Autodesk Fusion 360 part; units mm, degrees
note: some values were not read from the file. Chosen so that the rebuilt part matches the saved one: that a step has no effect.
(part 7 of 7)
  spline S315 degree 3 poles (62.2159, 94.3594) (61.6701, 95.351) (61.6701, 95.351) (61.5911, 95.6457) knots 0 0 0 0 1 1 1 1
  spline S316 degree 3 poles (61.5911, 95.6457) (61.8402, 95.8709) (62.0898, 96.0953) (62.3397, 96.3195) knots 0 0 0 0 1 1 1 1
  spline S317 degree 3 poles (62.3397, 96.3195) (62.4451, 96.4149) (62.4451, 96.4149) (62.5526, 96.5123) knots 0 0 0 0 1 1 1 1
  spline S318 degree 3 poles (62.5526, 96.5123) (63.3308, 97.2082) (64.2415, 97.7243) (65.322, 97.5831) knots 0 0 0 0 1 1 1 1
  spline S319 degree 3 poles (-22.0549, 83.1437) (-21.9278, 83.1778) (-21.8007, 83.2119) (-21.6697, 83.247) knots 0 0 0 0 1 1 1 1
  spline S320 degree 3 poles (-21.6697, 83.247) (-21.2763, 82.8034) (-21.2052, 82.1251) (-21.0547, 81.5621) knots 0 0 0 0 1 1 1 1
  spline S321 degree 3 poles (-21.0547, 81.5621) (-21.0162, 81.4183) (-20.9777, 81.2746) (-20.938, 81.1265) knots 0 0 0 0 1 1 1 1
  spline S322 degree 3 poles (-20.938, 81.1265) (-20.5691, 79.7113) (-20.212, 78.2272) (-20.2059, 76.7566) knots 0 0 0 0 1 1 1 1
  spline S323 degree 3 poles (-20.2059, 76.7566) (-21.5811, 76.4463) (-22.956, 76.389) (-24.3593, 76.332) knots 0 0 0 0 1 1 1 1
  spline S324 degree 3 poles (-24.3593, 76.332) (-24.1584, 77.2005) (-23.9104, 78.0286) (-23.5915, 78.8606) knots 0 0 0 0 1 1 1 1
  spline S325 degree 3 poles (-23.5915, 78.8606) (-23.3151, 79.5912) (-23.0456, 80.3225) (-22.7959, 81.0627) knots 0 0 0 0 1 1 1 1
  spline S326 degree 3 poles (-22.7959, 81.0627) (-22.7509, 81.195) (-22.706, 81.3273) (-22.6597, 81.4636) knots 0 0 0 0 1 1 1 1
  spline S327 degree 3 poles (-22.6597, 81.4636) (-22.5724, 81.7219) (-22.4863, 81.9806) (-22.4015, 82.2397) knots 0 0 0 0 1 1 1 1
  spline S328 degree 3 poles (-22.4015, 82.2397) (-22.3618, 82.3564) (-22.3221, 82.4731) (-22.2812, 82.5933) knots 0 0 0 0 1 1 1 1
  spline S329 degree 3 poles (-22.2812, 82.5933) (-22.2295, 82.7492) (-22.2295, 82.7492) (-22.1768, 82.9082) knots 0 0 0 0 1 1 1 1
  spline S330 degree 3 poles (-22.1768, 82.9082) (-22.1366, 82.9859) (-22.0964, 83.0636) (-22.0549, 83.1437) knots 0 0 0 0 1 1 1 1
  spline S331 degree 3 poles (61.5057, 102.6431) (61.936, 102.5114) (62.1851, 102.4146) (62.4827, 102.0789) knots 0 0 0 0 1 1 1 1
  spline S332 degree 3 poles (62.4827, 102.0789) (62.7043, 101.4281) (62.7203, 100.8901) (62.4367, 100.2599) knots 0 0 0 0 1 1 1 1
  spline S333 degree 3 poles (62.4367, 100.2599) (61.9549, 99.393) (61.2756, 98.5426) (60.3891, 98.0767) knots 0 0 0 0 1 1 1 1
  spline S334 degree 3 poles (60.3891, 98.0767) (60.05, 98.4814) (59.7123, 98.8872) (59.3749, 99.2933) knots 0 0 0 0 1 1 1 1
  spline S335 degree 3 poles (59.3749, 99.2933) (59.2784, 99.4084) (59.1819, 99.5235) (59.0825, 99.6421) knots 0 0 0 0 1 1 1 1
  spline S336 degree 3 poles (59.0825, 99.6421) (58.9907, 99.7528) (58.8989, 99.8635) (58.8044, 99.9776) knots 0 0 0 0 1 1 1 1
  spline S337 degree 3 poles (58.8044, 99.9776) (58.7194, 100.0795) (58.6344, 100.1815) (58.5468, 100.2865) knots 0 0 0 0 1 1 1 1
  spline S338 degree 3 poles (58.5468, 100.2865) (58.3477, 100.558) (58.3477, 100.558) (58.2445, 100.9433) knots 0 0 0 0 1 1 1 1
  spline S339 degree 3 poles (58.2445, 100.9433) (58.57, 101.1706) (58.8969, 101.3953) (59.2249, 101.619) knots 0 0 0 0 1 1 1 1
  spline S340 degree 3 poles (59.2249, 101.619) (59.361, 101.7145) (59.361, 101.7145) (59.4998, 101.812) knots 0 0 0 0 1 1 1 1
  spline S341 degree 3 poles (59.4998, 101.812) (60.1264, 102.2358) (60.7438, 102.5566) (61.5057, 102.6431) knots 0 0 0 0 1 1 1 1
extrude "Extrude6" cut sketch "Sketch107" against normal blind 0.4 contours S0 S1 S2 S3 S4 S5 S6 S7 S8 S9 S10 S11 S12 S13 S14 S15 S16 S17 S18 S19 S20 S21 S22 S23 S24 S25 S26 S27 S28 S29 S30 S31 S32 S33 S34 S35 S36 S37 S38 S39 S40 S41 S42 S43 S44 S45 S46 S47 S48 S49 S50 S51 S52 S53 S54 S65 S66 S67 S114 S115 S116 S117 S118 S119 S120 | S54 S55 S56 S57 S58 S59 S60 S61 S62 S63 S64 S65 S114 S115 S116 S117 S118 S119 S120 S121 S122 S123 S124 S125 S126 S127 S128 S129 S130 | S308 S309 S310 S311 S312 S313 S314 S315 S316 S317 S318 | S319 S320 S321 S322 S323 S324 S325 S326 S327 S328 S329 S330 | S331 S332 S333 S334 S335 S336 S337 S338 S339 S340 S341 bodies 2 in component "Component"
sketch "Sketch108" plane through (0, -33.2802, 118.858) normal (0, -0.26963, 0.962964) x (1, 0, 0)
  line L0 (-103.3594, -20.3608) -> (76.6406, -20.3608)
  line L1 (76.6406, -20.3608) -> (76.6406, 97.166)
  line L2 (76.6406, 97.166) -> (71.6406, 97.166)
  line L3 (71.6406, 97.166) -> (71.6406, 62.066)
  line L4 (71.6406, 62.066) -> (-98.3594, 62.066)
  line L5 (-98.3594, 62.066) -> (-98.3594, 97.166)
  line L6 (-98.3594, 97.166) -> (-103.3594, 97.166)
  line L7 (-103.3594, 97.166) -> (-103.3594, -20.3608)
  spline S0 degree 3 poles (-85.2606, 64.3178) (-39.3625, 64.3178) (6.5356, 64.3178) (53.8246, 64.3178) knots 0 0 0 0 1 1 1 1
  spline S1 degree 3 poles (53.8246, 64.3178) (53.8246, 35.1839) (53.8246, 6.05) (53.8246, -23.9668) knots 0 0 0 0 1 1 1 1
  spline S2 degree 3 poles (53.8246, -23.9668) (7.9265, -23.9668) (-37.9717, -23.9668) (-85.2606, -23.9668) knots 0 0 0 0 1 1 1 1
  spline S3 degree 3 poles (-85.2606, -23.9668) (-85.2606, 5.1671) (-85.2606, 34.3011) (-85.2606, 64.3178) knots 0 0 0 0 1 1 1 1
  spline S4 degree 3 poles (-40.7041, 45.5277) (-42.4517, 43.0465) (-42.7552, 40.6645) (-42.3514, 37.6845) knots 0 0 0 0 1 1 1 1
  spline S5 degree 3 poles (-42.3514, 37.6845) (-41.6687, 35.5957) (-40.6171, 34.2385) (-38.7448, 33.0915) knots 0 0 0 0 1 1 1 1
  spline S6 degree 3 poles (-38.7448, 33.0915) (-35.2679, 31.3825) (-32.3234, 31.0033) (-28.5415, 31.766) knots 0 0 0 0 1 1 1 1
  spline S7 degree 3 poles (-28.5415, 31.766) (-26.5081, 32.5567) (-24.9395, 33.4626) (-23.6094, 35.2184) knots 0 0 0 0 1 1 1 1
  spline S8 degree 3 poles (-23.6094, 35.2184) (-23.6767, 36.3127) (-23.6767, 36.3127) (-24.1026, 37.1913) knots 0 0 0 0 1 1 1 1
  spline S9 degree 3 poles (-24.1026, 37.1913) (-25.7404, 37.0008) (-26.8845, 36.8089) (-28.2949, 35.9274) knots 0 0 0 0 1 1 1 1
  spline S10 degree 3 poles (-28.2949, 35.9274) (-29.8328, 35.0431) (-30.7377, 34.9951) (-32.4872, 35.2184) knots 0 0 0 0 1 1 1 1
  spline S11 degree 3 poles (-32.4872, 35.2184) (-34.0338, 36.0963) (-34.3816, 36.4628) (-34.9532, 38.1777) knots 0 0 0 0 1 1 1 1
  spline S12 degree 3 poles (-34.9532, 38.1777) (-35.2257, 40.9021) (-34.6294, 42.6777) (-33.4601, 45.0749) knots 0 0 0 0 1 1 1 1
  spline S13 degree 3 poles (-33.4601, 45.0749) (-32.9256, 46.1286) (-32.9256, 46.1286) (-32.4872, 47.5487) knots 0 0 0 0 1 1 1 1
  spline S14 degree 3 poles (-32.4872, 47.5487) (-31.7786, 47.5888) (-31.0695, 47.6174) (-30.3602, 47.6412) knots 0 0 0 0 1 1 1 1
  spline S15 degree 3 poles (-30.3602, 47.6412) (-29.768, 47.6669) (-29.768, 47.6669) (-29.1638, 47.6932) knots 0 0 0 0 1 1 1 1
  spline S16 degree 3 poles (-29.1638, 47.6932) (-27.7795, 47.5139) (-27.4143, 47.1563) (-26.5686, 46.0691) knots 0 0 0 0 1 1 1 1
  spline S17 degree 3 poles (-26.5686, 46.0691) (-26.0526, 45.0944) (-25.5554, 44.1092) (-25.089, 43.1098) knots 0 0 0 0 1 1 1 1
  spline S18 degree 3 poles (-25.089, 43.1098) (-23.7295, 43.3552) (-23.7295, 43.3552) (-22.623, 44.0962) knots 0 0 0 0 1 1 1 1
  spline S19 degree 3 poles (-22.623, 44.0962) (-22.5874, 44.9278) (-22.5816, 45.7608) (-22.5921, 46.5931) knots 0 0 0 0 1 1 1 1
  spline S20 degree 3 poles (-22.5921, 46.5931) (-22.5966, 47.0464) (-22.601, 47.4997) (-22.6056, 47.9668) knots 0 0 0 0 1 1 1 1
  spline S21 degree 3 poles (-22.6056, 47.9668) (-22.6113, 48.3171) (-22.6171, 48.6674) (-22.623, 49.0283) knots 0 0 0 0 1 1 1 1
  spline S22 degree 3 poles (-22.623, 49.0283) (-29.2496, 52.7767) (-35.9767, 51.5009) (-40.7041, 45.5277) knots 0 0 0 0 1 1 1 1
  spline S23 degree 3 poles (-20.1569, 50.0147) (-19.9942, 49.5265) (-19.8314, 49.0382) (-19.6637, 48.5351) knots 0 0 0 0 1 1 1 1
  spline S24 degree 3 poles (-19.6637, 48.5351) (-19.5212, 45.3435) (-19.9211, 42.3152) (-20.4035, 39.1641) knots 0 0 0 0 1 1 1 1
  spline S25 degree 3 poles (-20.4035, 39.1641) (-20.4741, 38.6879) (-20.5447, 38.2117) (-20.6174, 37.7211) knots 0 0 0 0 1 1 1 1
  spline S26 degree 3 poles (-20.6174, 37.7211) (-20.7902, 36.5577) (-20.9655, 35.3947) (-21.1433, 34.232) knots 0 0 0 0 1 1 1 1
  spline S27 degree 3 poles (-21.1433, 34.232) (-21.4689, 34.232) (-21.7944, 34.232) (-22.1298, 34.232) knots 0 0 0 0 1 1 1 1
  spline S28 degree 3 poles (-22.1298, 34.232) (-22.4211, 33.2722) (-22.4211, 33.2722) (-22.623, 32.2592) knots 0 0 0 0 1 1 1 1
  spline S29 degree 3 poles (-22.623, 32.2592) (-22.0368, 31.5599) (-22.0368, 31.5599) (-20.3554, 31.7178) knots 0 0 0 0 1 1 1 1
  spline S30 degree 3 poles (-20.3554, 31.7178) (-19.6213, 31.7211) (-18.8873, 31.727) (-18.1532, 31.7351) knots 0 0 0 0 1 1 1 1
  spline S31 degree 3 poles (-18.1532, 31.7351) (-17.7791, 31.7374) (-17.4049, 31.7396) (-17.0194, 31.7419) knots 0 0 0 0 1 1 1 1
  spline S32 degree 3 poles (-17.0194, 31.7419) (-16.0924, 31.7477) (-15.1654, 31.7566) (-14.2384, 31.766) knots 0 0 0 0 1 1 1 1
  spline S33 degree 3 poles (-14.2384, 31.766) (-13.7776, 33.2507) (-13.7232, 33.673) (-14.2384, 35.2184) knots 0 0 0 0 1 1 1 1
  spline S34 degree 3 poles (-14.2384, 35.2184) (-14.0745, 37.1056) (-13.7051, 38.9641) (-13.3753, 40.8287) knots 0 0 0 0 1 1 1 1
  spline S35 degree 3 poles (-13.3753, 40.8287) (-13.2914, 41.3424) (-13.2074, 41.8561) (-13.121, 42.3854) knots 0 0 0 0 1 1 1 1
  spline S36 degree 3 poles (-13.121, 42.3854) (-13.0345, 42.8826) (-12.948, 43.3797) (-12.8589, 43.892) knots 0 0 0 0 1 1 1 1
  spline S37 degree 3 poles (-12.8589, 43.892) (-12.7809, 44.3449) (-12.7029, 44.7978) (-12.6225, 45.2645) knots 0 0 0 0 1 1 1 1
  spline S38 degree 3 poles (-12.6225, 45.2645) (-12.2264, 46.7045) (-11.5592, 47.7594) (-10.7859, 49.0283) knots 0 0 0 0 1 1 1 1
  spline S39 degree 3 poles (-10.7859, 49.0283) (-10.8877, 50.1397) (-10.8877, 50.1397) (-11.2791, 51.0012) knots 0 0 0 0 1 1 1 1
  spline S40 degree 3 poles (-11.2791, 51.0012) (-12.4815, 51.0278) (-13.6832, 51.0473) (-14.8857, 51.0628) knots 0 0 0 0 1 1 1 1
  spline S41 degree 3 poles (-14.8857, 51.0628) (-15.2262, 51.0711) (-15.5666, 51.0793) (-15.9174, 51.0879) knots 0 0 0 0 1 1 1 1
  spline S42 degree 3 poles (-15.9174, 51.0879) (-17.7754, 51.1058) (-18.5709, 51.0721) (-20.1569, 50.0147) knots 0 0 0 0 1 1 1 1
  spline S43 degree 3 poles (-5.613, 45.6895) (-7.6767, 42.5967) (-9.4221, 39.2931) (-11.1905, 36.0257) knots 0 0 0 0 1 1 1 1
  spline S44 degree 3 poles (-11.1905, 36.0257) (-14.2871, 30.4504) (-14.2871, 30.4504) (-17.1977, 28.8067) knots 0 0 0 0 1 1 1 1
  spline S45 degree 3 poles (-17.1977, 28.8067) (-19.8296, 28.0547) (-21.5351, 28.5063) (-24.1026, 29.2999) knots 0 0 0 0 1 1 1 1
  spline S46 degree 3 poles (-24.1026, 29.2999) (-25.706, 29.4242) (-25.706, 29.4242) (-27.0619, 29.2999) knots 0 0 0 0 1 1 1 1
  spline S47 degree 3 poles (-27.0619, 29.2999) (-27.7012, 28.7739) (-27.7012, 28.7739) (-27.5859, 27.5428) knots 0 0 0 0 1 1 1 1
  spline S48 degree 3 poles (-27.5859, 27.5428) (-27.5757, 27.1461) (-27.5655, 26.7494) (-27.5551, 26.3406) knots 0 0 0 0 1 1 1 1
  spline S49 degree 3 poles (-27.5551, 26.3406) (-24.4031, 24.4376) (-21.86, 23.7936) (-18.1841, 24.3678) knots 0 0 0 0 1 1 1 1
  spline S50 degree 3 poles (-18.1841, 24.3678) (-13.7607, 25.7268) (-10.6964, 28.7124) (-8.5145, 32.7312) knots 0 0 0 0 1 1 1 1
  spline S51 degree 3 poles (-8.5145, 32.7312) (-7.3022, 35.1114) (-7.3022, 35.1114) (-6.8402, 37.6845) knots 0 0 0 0 1 1 1 1
  spline S52 degree 3 poles (-6.8402, 37.6845) (-5.0499, 37.6845) (-3.2595, 37.6845) (-1.4149, 37.6845) knots 0 0 0 0 1 1 1 1
  spline S53 degree 3 poles (-1.4149, 37.6845) (-1.8002, 36.7212) (-2.1856, 35.7579) (-2.5709, 34.7946) knots 0 0 0 0 1 1 1 1
  spline S54 degree 3 poles (-2.5709, 34.7946) (-2.9909, 33.6085) (-2.9909, 33.6085) (-2.8946, 31.766) knots 0 0 0 0 1 1 1 1
  spline S55 degree 3 poles (-2.8946, 31.766) (-0.2904, 31.766) (2.3137, 31.766) (4.9968, 31.766) knots 0 0 0 0 1 1 1 1
  spline S56 degree 3 poles (4.9968, 31.766) (5.7135, 34.0374) (5.7135, 34.0374) (4.9968, 35.2184) knots 0 0 0 0 1 1 1 1
  spline S57 degree 3 poles (4.9968, 35.2184) (5.0969, 36.1135) (5.2375, 37.0043) (5.3975, 37.8906) knots 0 0 0 0 1 1 1 1
  spline S58 degree 3 poles (5.3975, 37.8906) (5.5368, 38.697) (5.5368, 38.697) (5.6788, 39.5196) knots 0 0 0 0 1 1 1 1
  spline S59 degree 3 poles (5.6788, 39.5196) (5.8801, 40.6501) (6.083, 41.7804) (6.2876, 42.9104) knots 0 0 0 0 1 1 1 1
  spline S60 degree 3 poles (6.2876, 42.9104) (6.7776, 45.7645) (7.1334, 48.1637) (6.4764, 51.0012) knots 0 0 0 0 1 1 1 1
  spline S61 degree 3 poles (6.4764, 51.0012) (1.4344, 51.5805) (-2.4821, 49.6847) (-5.613, 45.6895) knots 0 0 0 0 1 1 1 1
  spline S62 degree 3 poles (10.1485, 46.5025) (8.6042, 44.4949) (8.3133, 42.6425) (8.326, 40.1505) knots 0 0 0 0 1 1 1 1
  spline S63 degree 3 poles (8.326, 40.1505) (8.3234, 39.6521) (8.3209, 39.1536) (8.3183, 38.6401) knots 0 0 0 0 1 1 1 1
  spline S64 degree 3 poles (8.3183, 38.6401) (8.4873, 36.7705) (8.83, 35.3437) (10.1659, 33.9796) knots 0 0 0 0 1 1 1 1
  spline S65 degree 3 poles (10.1659, 33.9796) (13.1803, 31.9033) (16.0835, 30.8955) (19.7931, 31.2727) knots 0 0 0 0 1 1 1 1
  spline S66 degree 3 poles (19.7931, 31.2727) (23.0035, 32.1856) (26.0863, 33.5214) (28.1777, 36.2049) knots 0 0 0 0 1 1 1 1
  spline S67 degree 3 poles (28.1777, 36.2049) (29.8517, 39.3641) (30.5992, 42.1028) (29.6573, 45.5758) knots 0 0 0 0 1 1 1 1
  spline S68 degree 3 poles (29.6573, 45.5758) (28.1947, 48.3927) (26.2568, 49.9974) (23.2456, 51.0012) knots 0 0 0 0 1 1 1 1
  spline S69 degree 3 poles (23.2456, 51.0012) (17.48, 51.4823) (14.2014, 50.5648) (10.1485, 46.5025) knots 0 0 0 0 1 1 1 1
  spline S70 degree 3 poles (28.2702, 35.0951) (27.5731, 34.2643) (27.5731, 34.2643) (27.7769, 33.2148) knots 0 0 0 0 1 1 1 1
  spline S71 degree 3 poles (27.7769, 33.2148) (28.1455, 32.1669) (28.1455, 32.1669) (29.1641, 31.2727) knots 0 0 0 0 1 1 1 1
  spline S72 degree 3 poles (29.1641, 31.2727) (30.7951, 31.4157) (30.7951, 31.4157) (32.1234, 32.2592) knots 0 0 0 0 1 1 1 1
  spline S73 degree 3 poles (32.1234, 32.2592) (32.2467, 33.4715) (32.2467, 33.4715) (32.1234, 34.7252) knots 0 0 0 0 1 1 1 1
  spline S74 degree 3 poles (32.1234, 34.7252) (31.7978, 35.0507) (31.4723, 35.3763) (31.1369, 35.7116) knots 0 0 0 0 1 1 1 1
  spline S75 degree 3 poles (31.1369, 35.7116) (29.2538, 35.8983) (29.2538, 35.8983) (28.2702, 35.0951) knots 0 0 0 0 1 1 1 1
  spline S76 degree 3 poles (-73.2695, 21.4085) (-78.0088, 15.3054) (-81.4027, 7.6793) (-80.7004, -0.1694) knots 0 0 0 0 1 1 1 1
  spline S77 degree 3 poles (-80.7004, -0.1694) (-80.2348, -2.8721) (-79.3572, -4.9057) (-77.8625, -7.1976) knots 0 0 0 0 1 1 1 1
  spline S78 degree 3 poles (-77.8625, -7.1976) (-77.537, -7.1976) (-77.2115, -7.1976) (-76.8761, -7.1976) knots 0 0 0 0 1 1 1 1
  spline S79 degree 3 poles (-76.8761, -7.1976) (-76.7133, -7.6859) (-76.5506, -8.1742) (-76.3829, -8.6773) knots 0 0 0 0 1 1 1 1
  spline S80 degree 3 poles (-76.3829, -8.6773) (-73.4275, -10.6752) (-70.2981, -10.9696) (-66.8269, -10.8967) knots 0 0 0 0 1 1 1 1
  spline S81 degree 3 poles (-66.8269, -10.8967) (-66.3712, -10.8908) (-65.9155, -10.8848) (-65.446, -10.8787) knots 0 0 0 0 1 1 1 1
  spline S82 degree 3 poles (-65.446, -10.8787) (-62.0519, -10.78) (-59.1701, -10.3368) (-56.1613, -8.6773) knots 0 0 0 0 1 1 1 1
  spline S83 degree 3 poles (-56.1613, -8.6773) (-55.591, -8.3635) (-55.591, -8.3635) (-55.0091, -8.0434) knots 0 0 0 0 1 1 1 1
  spline S84 degree 3 poles (-55.0091, -8.0434) (-52.1188, -6.2727) (-49.3165, -4.0019) (-47.2835, -1.2791) knots 0 0 0 0 1 1 1 1
  spline S85 degree 3 poles (-47.2835, -1.2791) (-46.8889, 0.2825) (-46.8889, 0.2825) (-46.7903, 1.6801) knots 0 0 0 0 1 1 1 1
  spline S86 degree 3 poles (-46.7903, 1.6801) (-47.1158, 1.8429) (-47.4413, 2.0057) (-47.7767, 2.1734) knots 0 0 0 0 1 1 1 1
  spline S87 degree 3 poles (-47.7767, 2.1734) (-49.2164, 1.417) (-50.5879, 0.5928) (-51.9719, -0.259) knots 0 0 0 0 1 1 1 1
  spline S88 degree 3 poles (-51.9719, -0.259) (-56.0111, -2.6756) (-60.4601, -3.5933) (-65.1142, -2.5121) knots 0 0 0 0 1 1 1 1
  spline S89 degree 3 poles (-65.1142, -2.5121) (-67.4944, -1.5955) (-69.3008, -0.1484) (-70.4509, 2.1425) knots 0 0 0 0 1 1 1 1
  spline S90 degree 3 poles (-70.4509, 2.1425) (-72.1941, 6.683) (-71.7953, 11.0244) (-70.131, 15.5266) knots 0 0 0 0 1 1 1 1
  spline S91 degree 3 poles (-70.131, 15.5266) (-68.079, 20.0605) (-65.1634, 23.3862) (-60.6618, 25.5392) knots 0 0 0 0 1 1 1 1
  spline S92 degree 3 poles (-60.6618, 25.5392) (-58.0055, 26.0704) (-55.3363, 26.4761) (-52.8937, 25.1384) knots 0 0 0 0 1 1 1 1
  spline S93 degree 3 poles (-52.8937, 25.1384) (-51.8694, 23.2295) (-51.918, 21.5549) (-52.2156, 19.4357) knots 0 0 0 0 1 1 1 1
  spline S94 degree 3 poles (-52.2156, 19.4357) (-53.0965, 16.7929) (-54.2667, 14.4981) (-56.5928, 12.8698) knots 0 0 0 0 1 1 1 1
  spline S95 degree 3 poles (-56.5928, 12.8698) (-57.9576, 12.4283) (-59.1759, 12.466) (-60.6001, 12.5308) knots 0 0 0 0 1 1 1 1
  spline S96 degree 3 poles (-60.6001, 12.5308) (-60.7629, 12.8563) (-60.9257, 13.1818) (-61.0934, 13.5172) knots 0 0 0 0 1 1 1 1
  spline S97 degree 3 poles (-61.0934, 13.5172) (-60.5542, 13.6291) (-60.0151, 13.741) (-59.4596, 13.8563) knots 0 0 0 0 1 1 1 1
  spline S98 degree 3 poles (-59.4596, 13.8563) (-57.6146, 14.3445) (-57.6146, 14.3445) (-56.6545, 15.6442) knots 0 0 0 0 1 1 1 1
  spline S99 degree 3 poles (-56.6545, 15.6442) (-56.0817, 17.1835) (-56.1144, 17.8985) (-56.6545, 19.4357) knots 0 0 0 0 1 1 1 1
  spline S100 degree 3 poles (-56.6545, 19.4357) (-57.6036, 20.5897) (-57.6036, 20.5897) (-59.2746, 20.6071) knots 0 0 0 0 1 1 1 1
  spline S101 degree 3 poles (-59.2746, 20.6071) (-61.4236, 20.3885) (-62.1051, 20.0248) (-63.5594, 18.4493) knots 0 0 0 0 1 1 1 1
  spline S102 degree 3 poles (-63.5594, 18.4493) (-64.8482, 16.0939) (-65.3797, 14.221) (-65.039, 11.5443) knots 0 0 0 0 1 1 1 1
  spline S103 degree 3 poles (-65.039, 11.5443) (-64.1177, 9.5482) (-63.2171, 8.503) (-61.2167, 7.6603) knots 0 0 0 0 1 1 1 1
  spline S104 degree 3 poles (-61.2167, 7.6603) (-57.452, 6.4913) (-54.2797, 7.0503) (-50.7359, 8.5851) knots 0 0 0 0 1 1 1 1
  spline S105 degree 3 poles (-50.7359, 8.5851) (-47.2755, 10.515) (-45.0132, 13.1743) (-43.831, 16.9697) knots 0 0 0 0 1 1 1 1
  spline S106 degree 3 poles (-43.831, 16.9697) (-43.3947, 20.5243) (-43.7109, 23.3885) (-45.8038, 26.3406) knots 0 0 0 0 1 1 1 1
  spline S107 degree 3 poles (-45.8038, 26.3406) (-47.5426, 28.5336) (-48.9701, 29.5622) (-51.7224, 30.2863) knots 0 0 0 0 1 1 1 1
  spline S108 degree 3 poles (-51.7224, 30.2863) (-60.4832, 31.1736) (-67.4326, 28.065) (-73.2695, 21.4085) knots 0 0 0 0 1 1 1 1
  spline S109 degree 3 poles (-35.0457, 27.1113) (-35.6002, 26.9315) (-35.6002, 26.9315) (-36.166, 26.7481) knots 0 0 0 0 1 1 1 1
  spline S110 degree 3 poles (-36.166, 26.7481) (-37.0783, 26.4518) (-37.9887, 26.1501) (-38.8989, 25.8474) knots 0 0 0 0 1 1 1 1
  spline S111 degree 3 poles (-38.8989, 25.8474) (-38.8772, 25.3569) (-38.8556, 24.8664) (-38.8333, 24.3611) knots 0 0 0 0 1 1 1 1
  spline S112 degree 3 poles (-38.8333, 24.3611) (-38.9025, 22.2864) (-39.3281, 20.5171) (-39.9489, 18.5572) knots 0 0 0 0 1 1 1 1
  spline S113 degree 3 poles (-39.9489, 18.5572) (-40.0593, 18.1962) (-40.1698, 17.8352) (-40.2836, 17.4633) knots 0 0 0 0 1 1 1 1
  spline S114 degree 3 poles (-40.2836, 17.4633) (-40.6385, 16.3105) (-41.001, 15.1603) (-41.3649, 14.0104) knots 0 0 0 0 1 1 1 1
  spline S115 degree 3 poles (-41.3649, 14.0104) (-41.4824, 13.6347) (-41.5999, 13.2591) (-41.721, 12.872) knots 0 0 0 0 1 1 1 1
  spline S116 degree 3 poles (-41.721, 12.872) (-42.436, 10.5875) (-43.169, 8.3096) (-43.9171, 6.0357) knots 0 0 0 0 1 1 1 1
  spline S117 degree 3 poles (-43.9171, 6.0357) (-44.17, 5.2631) (-44.4199, 4.4896) (-44.667, 3.7151) knots 0 0 0 0 1 1 1 1
  spline S118 degree 3 poles (-44.667, 3.7151) (-47.166, -4.1117) (-47.166, -4.1117) (-49.6042, -7.3238) knots 0 0 0 0 1 1 1 1
  spline S119 degree 3 poles (-49.6042, -7.3238) (-50.2742, -8.2265) (-50.7538, -9.1404) (-51.2292, -10.1569) knots 0 0 0 0 1 1 1 1
  spline S120 degree 3 poles (-51.2292, -10.1569) (-50.7279, -10.7681) (-50.7279, -10.7681) (-49.6839, -10.7061) knots 0 0 0 0 1 1 1 1
  spline S121 degree 3 poles (-49.6839, -10.7061) (-49.2319, -10.7035) (-48.7799, -10.7009) (-48.3142, -10.6983) knots 0 0 0 0 1 1 1 1
  spline S122 degree 3 poles (-48.3142, -10.6983) (-47.8262, -10.6967) (-47.3383, -10.6951) (-46.8355, -10.6935) knots 0 0 0 0 1 1 1 1
  spline S123 degree 3 poles (-46.8355, -10.6935) (-46.0654, -10.6873) (-46.0654, -10.6873) (-45.2798, -10.6809) knots 0 0 0 0 1 1 1 1
  spline S124 degree 3 poles (-45.2798, -10.6809) (-44.7645, -10.6787) (-44.2492, -10.6765) (-43.7183, -10.6742) knots 0 0 0 0 1 1 1 1
  spline S125 degree 3 poles (-43.7183, -10.6742) (-42.4406, -10.6684) (-41.163, -10.6602) (-39.8853, -10.6501) knots 0 0 0 0 1 1 1 1
  spline S126 degree 3 poles (-39.8853, -10.6501) (-39.262, -9.1699) (-39.262, -9.1699) (-39.6701, -7.5708) knots 0 0 0 0 1 1 1 1
  spline S127 degree 3 poles (-39.6701, -7.5708) (-39.9162, -5.4522) (-39.5803, -4.2201) (-38.8893, -2.2135) knots 0 0 0 0 1 1 1 1
  spline S128 degree 3 poles (-38.8893, -2.2135) (-38.7814, -1.8947) (-38.6736, -1.5758) (-38.5625, -1.2473) knots 0 0 0 0 1 1 1 1
  spline S129 degree 3 poles (-38.5625, -1.2473) (-38.2192, -0.2381) (-37.8655, 0.7671) (-37.5117, 1.7726) knots 0 0 0 0 1 1 1 1
  spline S130 degree 3 poles (-37.5117, 1.7726) (-37.2796, 2.4528) (-37.0481, 3.1332) (-36.8172, 3.8139) knots 0 0 0 0 1 1 1 1
  spline S131 degree 3 poles (-36.8172, 3.8139) (-34.7674, 9.8031) (-34.7674, 9.8031) (-33.9668, 11.0511) knots 0 0 0 0 1 1 1 1
  spline S132 degree 3 poles (-33.9668, 11.0511) (-32.4255, 11.421) (-32.4255, 11.421) (-31.0075, 11.5443) knots 0 0 0 0 1 1 1 1
  spline S133 degree 3 poles (-31.0075, 11.5443) (-31.2308, 7.3201) (-32.5865, 3.5436) (-33.9668, -0.416) knots 0 0 0 0 1 1 1 1
  spline S134 degree 3 poles (-33.9668, -0.416) (-34.3116, -1.4157) (-34.6551, -2.4159) (-34.997, -3.4167) knots 0 0 0 0 1 1 1 1
  spline S135 degree 3 poles (-34.997, -3.4167) (-35.3061, -4.3197) (-35.6189, -5.2214) (-35.9319, -6.1231) knots 0 0 0 0 1 1 1 1
  spline S136 degree 3 poles (-35.9319, -6.1231) (-36.3634, -7.4734) (-36.7315, -8.7534) (-36.9261, -10.1569) knots 0 0 0 0 1 1 1 1
  spline S137 degree 3 poles (-36.9261, -10.1569) (-36.4354, -10.7569) (-36.4354, -10.7569) (-35.4714, -10.7061) knots 0 0 0 0 1 1 1 1
  spline S138 degree 3 poles (-35.4714, -10.7061) (-35.0607, -10.7035) (-34.65, -10.7009) (-34.2269, -10.6983) knots 0 0 0 0 1 1 1 1
  spline S139 degree 3 poles (-34.2269, -10.6983) (-33.5617, -10.6959) (-33.5617, -10.6959) (-32.8831, -10.6935) knots 0 0 0 0 1 1 1 1
  spline S140 degree 3 poles (-32.8831, -10.6935) (-32.4167, -10.6893) (-31.9504, -10.6852) (-31.4699, -10.6809) knots 0 0 0 0 1 1 1 1
  spline S141 degree 3 poles (-31.4699, -10.6809) (-30.7675, -10.6776) (-30.7675, -10.6776) (-30.051, -10.6742) knots 0 0 0 0 1 1 1 1
  spline S142 degree 3 poles (-30.051, -10.6742) (-28.8902, -10.6684) (-27.7294, -10.6602) (-26.5686, -10.6501) knots 0 0 0 0 1 1 1 1
  spline S143 degree 3 poles (-26.5686, -10.6501) (-26.5686, -9.9991) (-26.5686, -9.348) (-26.5686, -8.6773) knots 0 0 0 0 1 1 1 1
  spline S144 degree 3 poles (-26.5686, -8.6773) (-26.8942, -8.6773) (-27.2197, -8.6773) (-27.5551, -8.6773) knots 0 0 0 0 1 1 1 1
  spline S145 degree 3 poles (-27.5551, -8.6773) (-26.7835, -3.9316) (-25.2175, 0.5142) (-23.6595, 5.0498) knots 0 0 0 0 1 1 1 1
  spline S146 degree 3 poles (-23.6595, 5.0498) (-22.1892, 9.4421) (-22.1892, 9.4421) (-22.1298, 14.0104) knots 0 0 0 0 1 1 1 1
  spline S147 degree 3 poles (-22.1298, 14.0104) (-23.0521, 15.2095) (-23.7482, 15.806) (-25.089, 16.4764) knots 0 0 0 0 1 1 1 1
  spline S148 degree 3 poles (-25.089, 16.4764) (-25.8785, 16.5365) (-26.6708, 16.563) (-27.4626, 16.5689) knots 0 0 0 0 1 1 1 1
  spline S149 degree 3 poles (-27.4626, 16.5689) (-28.093, 16.5794) (-28.093, 16.5794) (-28.7361, 16.5901) knots 0 0 0 0 1 1 1 1
  spline S150 degree 3 poles (-28.7361, 16.5901) (-30.1451, 16.4655) (-31.205, 16.0724) (-32.4872, 15.49) knots 0 0 0 0 1 1 1 1
  spline S151 degree 3 poles (-32.4872, 15.49) (-32.415, 15.7584) (-32.3429, 16.0268) (-32.2686, 16.3033) knots 0 0 0 0 1 1 1 1
  spline S152 degree 3 poles (-32.2686, 16.3033) (-31.9393, 17.532) (-31.6121, 18.7613) (-31.285, 19.9906) knots 0 0 0 0 1 1 1 1
  spline S153 degree 3 poles (-31.285, 19.9906) (-31.1715, 20.4127) (-31.058, 20.8349) (-30.9411, 21.2698) knots 0 0 0 0 1 1 1 1
  spline S154 degree 3 poles (-30.9411, 21.2698) (-30.3637, 23.4452) (-29.8462, 25.5883) (-29.5279, 27.8203) knots 0 0 0 0 1 1 1 1
  spline S155 degree 3 poles (-29.5279, 27.8203) (-31.5851, 28.506) (-33.0702, 27.7721) (-35.0457, 27.1113) knots 0 0 0 0 1 1 1 1
  spline S156 degree 3 poles (11.9942, 16.5381) (10.1757, 15.7768) (8.349, 15.1203) (6.4764, 14.5036) knots 0 0 0 0 1 1 1 1
  spline S157 degree 3 poles (6.4764, 14.5036) (6.4331, 14.0568) (6.3898, 13.61) (6.3452, 13.1497) knots 0 0 0 0 1 1 1 1
  spline S158 degree 3 poles (6.3452, 13.1497) (5.8438, 8.7082) (4.9224, 4.7444) (3.4168, 0.5177) knots 0 0 0 0 1 1 1 1
  spline S159 degree 3 poles (3.4168, 0.5177) (3.0796, -0.4331) (2.7575, -1.3882) (2.4364, -2.3445) knots 0 0 0 0 1 1 1 1
  spline S160 degree 3 poles (2.4364, -2.3445) (0.8019, -7.0318) (0.8019, -7.0318) (-1.4149, -8.6773) knots 0 0 0 0 1 1 1 1
  spline S161 degree 3 poles (-1.4149, -8.6773) (-1.4149, -9.3283) (-1.4149, -9.9793) (-1.4149, -10.6501) knots 0 0 0 0 1 1 1 1
  spline S162 degree 3 poles (-1.4149, -10.6501) (2.1658, -10.6501) (5.7465, -10.6501) (9.4357, -10.6501) knots 0 0 0 0 1 1 1 1
  spline S163 degree 3 poles (9.4357, -10.6501) (9.5184, -8.7959) (9.5184, -8.7959) (9.1347, -7.5183) knots 0 0 0 0 1 1 1 1
  spline S164 degree 3 poles (9.1347, -7.5183) (8.8833, -5.8084) (9.2765, -4.692) (9.8133, -3.0535) knots 0 0 0 0 1 1 1 1
  spline S165 degree 3 poles (9.8133, -3.0535) (10.0085, -2.4518) (10.2037, -1.85) (10.4048, -1.23) knots 0 0 0 0 1 1 1 1
  spline S166 degree 3 poles (10.4048, -1.23) (10.509, -0.919) (10.6132, -0.608) (10.7205, -0.2875) knots 0 0 0 0 1 1 1 1
  spline S167 degree 3 poles (10.7205, -0.2875) (11.0364, 0.6564) (11.3436, 1.6028) (11.6494, 2.55) knots 0 0 0 0 1 1 1 1
  spline S168 degree 3 poles (11.6494, 2.55) (14.3196, 10.6853) (14.3196, 10.6853) (17.3271, 12.5308) knots 0 0 0 0 1 1 1 1
  spline S169 degree 3 poles (17.3271, 12.5308) (19.2074, 12.9007) (19.2074, 12.9007) (20.7795, 13.024) knots 0 0 0 0 1 1 1 1
  spline S170 degree 3 poles (20.7795, 13.024) (20.7795, 12.5357) (20.7795, 12.0474) (20.7795, 11.5443) knots 0 0 0 0 1 1 1 1
  spline S171 degree 3 poles (20.7795, 11.5443) (20.4744, 11.4935) (20.1692, 11.4426) (19.8548, 11.3902) knots 0 0 0 0 1 1 1 1
  spline S172 degree 3 poles (19.8548, 11.3902) (18.6265, 11.1127) (18.6265, 11.1127) (17.8203, 9.5715) knots 0 0 0 0 1 1 1 1
  spline S173 degree 3 poles (17.8203, 9.5715) (17.9768, 7.7765) (17.9768, 7.7765) (18.3135, 6.119) knots 0 0 0 0 1 1 1 1
  spline S174 degree 3 poles (18.3135, 6.119) (19.9073, 5.4519) (20.8892, 5.0434) (22.5982, 5.4409) knots 0 0 0 0 1 1 1 1
  spline S175 degree 3 poles (22.5982, 5.4409) (24.1425, 6.3591) (24.9213, 7.3085) (25.5575, 8.9858) knots 0 0 0 0 1 1 1 1
  spline S176 degree 3 poles (25.5575, 8.9858) (25.8645, 11.1348) (26.0149, 12.8819) (25.0643, 14.8735) knots 0 0 0 0 1 1 1 1
  spline S177 degree 3 poles (25.0643, 14.8735) (24.7896, 15.2397) (24.515, 15.6059) (24.232, 15.9832) knots 0 0 0 0 1 1 1 1
  spline S178 degree 3 poles (24.232, 15.9832) (23.9421, 16.4257) (23.9421, 16.4257) (23.6463, 16.8772) knots 0 0 0 0 1 1 1 1
  spline S179 degree 3 poles (23.6463, 16.8772) (22.1472, 17.8594) (20.5158, 17.7222) (18.8067, 17.4629) knots 0 0 0 0 1 1 1 1
  spline S180 degree 3 poles (18.8067, 17.4629) (17.3638, 16.7966) (17.3638, 16.7966) (16.3406, 15.9832) knots 0 0 0 0 1 1 1 1
  spline S181 degree 3 poles (16.3406, 15.9832) (16.0965, 16.7157) (16.0965, 16.7157) (15.8474, 17.4629) knots 0 0 0 0 1 1 1 1
  spline S182 degree 3 poles (15.8474, 17.4629) (14.2647, 17.4629) (13.439, 17.1462) (11.9942, 16.5381) knots 0 0 0 0 1 1 1 1
  spline S183 degree 3 poles (-0.0894, 16.7539) (-2.005, 16.2153) (-3.878, 15.757) (-5.8538, 15.49) knots 0 0 0 0 1 1 1 1
  spline S184 degree 3 poles (-5.8538, 15.49) (-5.8299, 15.1785) (-5.8059, 14.867) (-5.7812, 14.546) knots 0 0 0 0 1 1 1 1
  spline S185 degree 3 poles (-5.7812, 14.546) (-5.6074, 10.43) (-6.5886, 7.0269) (-7.9191, 3.1598) knots 0 0 0 0 1 1 1 1
  spline S186 degree 3 poles (-7.9191, 3.1598) (-8.2057, 2.2624) (-8.2057, 2.2624) (-8.4981, 1.3468) knots 0 0 0 0 1 1 1 1
  spline S187 degree 3 poles (-8.4981, 1.3468) (-8.6904, 0.7753) (-8.8827, 0.2037) (-9.0809, -0.3852) knots 0 0 0 0 1 1 1 1
  spline S188 degree 3 poles (-9.0809, -0.3852) (-9.2539, -0.9008) (-9.427, -1.4164) (-9.6053, -1.9477) knots 0 0 0 0 1 1 1 1
  spline S189 degree 3 poles (-9.6053, -1.9477) (-10.4333, -3.5188) (-11.1346, -4.043) (-12.7588, -4.7316) knots 0 0 0 0 1 1 1 1
  spline S190 degree 3 poles (-12.7588, -4.7316) (-13.4912, -4.4875) (-13.4912, -4.4875) (-14.2384, -4.2384) knots 0 0 0 0 1 1 1 1
  spline S191 degree 3 poles (-14.2384, -4.2384) (-13.9674, -1.5553) (-13.4816, 0.7977) (-12.6181, 3.3678) knots 0 0 0 0 1 1 1 1
  spline S192 degree 3 poles (-12.6181, 3.3678) (-12.5093, 3.697) (-12.4006, 4.0261) (-12.2885, 4.3651) knots 0 0 0 0 1 1 1 1
  spline S193 degree 3 poles (-12.2885, 4.3651) (-11.9452, 5.4031) (-11.5973, 6.4393) (-11.2483, 7.4754) knots 0 0 0 0 1 1 1 1
  spline S194 degree 3 poles (-11.2483, 7.4754) (-10.8978, 8.5185) (-10.5485, 9.562) (-10.2028, 10.6067) knots 0 0 0 0 1 1 1 1
  spline S195 degree 3 poles (-10.2028, 10.6067) (-9.8908, 11.5494) (-9.5745, 12.4907) (-9.258, 13.4319) knots 0 0 0 0 1 1 1 1
  spline S196 degree 3 poles (-9.258, 13.4319) (-8.7232, 15.0419) (-8.7232, 15.0419) (-8.8131, 16.9697) knots 0 0 0 0 1 1 1 1
  spline S197 degree 3 poles (-8.8131, 16.9697) (-12.2384, 17.2086) (-15.3723, 16.325) (-18.6773, 15.49) knots 0 0 0 0 1 1 1 1
  spline S198 degree 3 poles (-18.6773, 15.49) (-18.54, 14.9324) (-18.4026, 14.3749) (-18.2611, 13.8004) knots 0 0 0 0 1 1 1 1
  spline S199 degree 3 poles (-18.2611, 13.8004) (-17.8308, 9.9298) (-19.6212, 6.1665) (-20.8967, 2.5741) knots 0 0 0 0 1 1 1 1
  spline S200 degree 3 poles (-20.8967, 2.5741) (-21.2967, 1.4397) (-21.6938, 0.3047) (-22.0829, -0.8335) knots 0 0 0 0 1 1 1 1
  spline S201 degree 3 poles (-22.0829, -0.8335) (-22.3238, -1.5379) (-22.571, -2.2402) (-22.8254, -2.9399) knots 0 0 0 0 1 1 1 1
  spline S202 degree 3 poles (-22.8254, -2.9399) (-23.5469, -5.0416) (-23.7315, -6.5319) (-23.1162, -8.6773) knots 0 0 0 0 1 1 1 1
  spline S203 degree 3 poles (-23.1162, -8.6773) (-21.9924, -10.0632) (-21.3668, -10.5756) (-19.6637, -11.1433) knots 0 0 0 0 1 1 1 1
  spline S204 degree 3 poles (-19.6637, -11.1433) (-17.473, -11.2547) (-15.6495, -11.1836) (-13.5294, -10.6193) knots 0 0 0 0 1 1 1 1
  spline S205 degree 3 poles (-13.5294, -10.6193) (-12.9496, -10.4667) (-12.3697, -10.3141) (-11.7723, -10.1569) knots 0 0 0 0 1 1 1 1
  spline S206 degree 3 poles (-11.7723, -10.1569) (-11.5282, -10.401) (-11.5282, -10.401) (-11.2791, -10.6501) knots 0 0 0 0 1 1 1 1
  spline S207 degree 3 poles (-11.2791, -10.6501) (-9.8672, -10.6862) (-8.4675, -10.6957) (-7.056, -10.6809) knots 0 0 0 0 1 1 1 1
  spline S208 degree 3 poles (-7.056, -10.6809) (-6.4595, -10.6776) (-6.4595, -10.6776) (-5.8509, -10.6742) knots 0 0 0 0 1 1 1 1
  spline S209 degree 3 poles (-5.8509, -10.6742) (-4.8655, -10.6684) (-3.88, -10.6595) (-2.8946, -10.6501) knots 0 0 0 0 1 1 1 1
  spline S210 degree 3 poles (-2.8946, -10.6501) (-2.7318, -9.9991) (-2.569, -9.348) (-2.4013, -8.6773) knots 0 0 0 0 1 1 1 1
  spline S211 degree 3 poles (-2.4013, -8.6773) (-2.7269, -8.6773) (-3.0524, -8.6773) (-3.3878, -8.6773) knots 0 0 0 0 1 1 1 1
  spline S212 degree 3 poles (-3.3878, -8.6773) (-2.3863, -5.0562) (-1.3369, -1.4604) (-0.1607, 2.1078) knots 0 0 0 0 1 1 1 1
  spline S213 degree 3 poles (-0.1607, 2.1078) (-0.0008, 2.5939) (-0.0008, 2.5939) (0.1623, 3.0898) knots 0 0 0 0 1 1 1 1
  spline S214 degree 3 poles (0.1623, 3.0898) (0.5995, 4.4162) (1.0381, 5.742) (1.4811, 7.0664) knots 0 0 0 0 1 1 1 1
  spline S215 degree 3 poles (1.4811, 7.0664) (3.201, 12.1636) (3.201, 12.1636) (4.0104, 17.4629) knots 0 0 0 0 1 1 1 1
  spline S216 degree 3 poles (4.0104, 17.4629) (2.4787, 17.4629) (1.3767, 17.1777) (-0.0894, 16.7539) knots 0 0 0 0 1 1 1 1
  spline S217 degree 3 poles (42.8815, 16.4764) (42.3269, 16.3353) (42.3269, 16.3353) (41.7612, 16.1913) knots 0 0 0 0 1 1 1 1
  spline S218 degree 3 poles (41.7612, 16.1913) (40.8498, 15.9591) (39.939, 15.7248) (39.0283, 15.49) knots 0 0 0 0 1 1 1 1
  spline S219 degree 3 poles (39.0283, 15.49) (39.1008, 14.627) (39.1008, 14.627) (39.1747, 13.7464) knots 0 0 0 0 1 1 1 1
  spline S220 degree 3 poles (39.1747, 13.7464) (39.1722, 10.4816) (38.0728, 7.502) (37.0295, 4.4488) knots 0 0 0 0 1 1 1 1
  spline S221 degree 3 poles (37.0295, 4.4488) (36.6833, 3.4305) (36.3526, 2.4081) (36.0228, 1.3844) knots 0 0 0 0 1 1 1 1
  spline S222 degree 3 poles (36.0228, 1.3844) (35.8054, 0.7332) (35.587, 0.0824) (35.3678, -0.5682) knots 0 0 0 0 1 1 1 1
  spline S223 degree 3 poles (35.3678, -0.5682) (35.1715, -1.1547) (34.9752, -1.7411) (34.7729, -2.3454) knots 0 0 0 0 1 1 1 1
  spline S224 degree 3 poles (34.7729, -2.3454) (34.0962, -3.7452) (34.0962, -3.7452) (33.0997, -4.4485) knots 0 0 0 0 1 1 1 1
  spline S225 degree 3 poles (33.0997, -4.4485) (31.9333, -4.7867) (31.2817, -4.6424) (30.1505, -4.2384) knots 0 0 0 0 1 1 1 1
  spline S226 degree 3 poles (30.1505, -4.2384) (30.441, -1.7623) (30.9722, 0.4342) (31.7708, 2.8091) knots 0 0 0 0 1 1 1 1
  spline S227 degree 3 poles (31.7708, 2.8091) (31.994, 3.4834) (32.2172, 4.1577) (32.4403, 4.8321) knots 0 0 0 0 1 1 1 1
  spline S228 degree 3 poles (32.4403, 4.8321) (32.791, 5.88) (33.143, 6.9275) (33.4957, 7.9748) knots 0 0 0 0 1 1 1 1
  spline S229 degree 3 poles (33.4957, 7.9748) (33.8383, 8.9954) (34.1764, 10.0174) (34.5143, 11.0396) knots 0 0 0 0 1 1 1 1
  spline S230 degree 3 poles (34.5143, 11.0396) (34.7178, 11.6452) (34.9213, 12.2509) (35.1309, 12.8749) knots 0 0 0 0 1 1 1 1
  spline S231 degree 3 poles (35.1309, 12.8749) (35.5313, 14.3404) (35.6741, 15.4648) (35.5758, 16.9697) knots 0 0 0 0 1 1 1 1
  spline S232 degree 3 poles (35.5758, 16.9697) (30.8181, 16.625) (30.8181, 16.625) (26.2048, 15.49) knots 0 0 0 0 1 1 1 1
  spline S233 degree 3 poles (26.2048, 15.49) (25.5493, 14.4416) (25.5493, 14.4416) (26.0796, 12.9296) knots 0 0 0 0 1 1 1 1
  spline S234 degree 3 poles (26.0796, 12.9296) (26.5546, 9.5501) (24.9191, 6.3123) (23.7696, 3.1906) knots 0 0 0 0 1 1 1 1
  spline S235 degree 3 poles (23.7696, 3.1906) (21.5359, -2.5805) (21.5359, -2.5805) (21.2727, -8.6773) knots 0 0 0 0 1 1 1 1
  spline S236 degree 3 poles (21.2727, -8.6773) (22.9192, -10.4572) (24.3727, -11.0936) (26.7905, -11.2358) knots 0 0 0 0 1 1 1 1
  spline S237 degree 3 poles (26.7905, -11.2358) (28.2858, -11.1623) (29.4078, -10.9968) (30.8287, -10.6193) knots 0 0 0 0 1 1 1 1
  spline S238 degree 3 poles (30.8287, -10.6193) (31.4187, -10.4667) (32.0087, -10.3141) (32.6166, -10.1569) knots 0 0 0 0 1 1 1 1
  spline S239 degree 3 poles (32.6166, -10.1569) (32.8607, -10.401) (32.8607, -10.401) (33.1098, -10.6501) knots 0 0 0 0 1 1 1 1
  spline S240 degree 3 poles (33.1098, -10.6501) (33.772, -10.6927) (34.4364, -10.7029) (35.1, -10.6983) knots 0 0 0 0 1 1 1 1
  spline S241 degree 3 poles (35.1, -10.6983) (35.4989, -10.6967) (35.8979, -10.6951) (36.3089, -10.6935) knots 0 0 0 0 1 1 1 1
  spline S242 degree 3 poles (36.3089, -10.6935) (36.9379, -10.6873) (36.9379, -10.6873) (37.5795, -10.6809) knots 0 0 0 0 1 1 1 1
  spline S243 degree 3 poles (37.5795, -10.6809) (38.0007, -10.6787) (38.4219, -10.6765) (38.8559, -10.6742) knots 0 0 0 0 1 1 1 1
  spline S244 degree 3 poles (38.8559, -10.6742) (39.8998, -10.6684) (40.9437, -10.6595) (41.9876, -10.6501) knots 0 0 0 0 1 1 1 1
  spline S245 degree 3 poles (41.9876, -10.6501) (41.8528, -10.0849) (41.718, -9.5197) (41.5791, -8.9374) knots 0 0 0 0 1 1 1 1
  spline S246 degree 3 poles (41.5791, -8.9374) (41.1632, -5.1669) (42.8338, -1.5963) (44.0837, 1.8959) knots 0 0 0 0 1 1 1 1
  spline S247 degree 3 poles (44.0837, 1.8959) (44.3357, 2.6178) (44.5868, 3.3399) (44.837, 4.0624) knots 0 0 0 0 1 1 1 1
  spline S248 degree 3 poles (44.837, 4.0624) (45.2011, 5.1127) (45.5655, 6.1629) (45.932, 7.2124) knots 0 0 0 0 1 1 1 1
  spline S249 degree 3 poles (45.932, 7.2124) (47.8158, 12.2184) (47.8158, 12.2184) (48.3993, 17.4629) knots 0 0 0 0 1 1 1 1
  spline S250 degree 3 poles (48.3993, 17.4629) (46.4739, 17.4629) (44.7322, 16.9549) (42.8815, 16.4764) knots 0 0 0 0 1 1 1 1
  spline S251 degree 3 poles (44.4536, -4.7316) (44.1281, -5.7081) (43.8026, -6.6847) (43.4672, -7.6909) knots 0 0 0 0 1 1 1 1
  spline S252 degree 3 poles (43.4672, -7.6909) (44.1182, -8.3419) (44.7693, -8.9929) (45.44, -9.6637) knots 0 0 0 0 1 1 1 1
  spline S253 degree 3 poles (45.44, -9.6637) (47.2613, -9.1531) (47.2613, -9.1531) (48.3993, -7.7525) knots 0 0 0 0 1 1 1 1
  spline S254 degree 3 poles (48.3993, -7.7525) (48.4774, -6.6539) (48.4774, -6.6539) (47.8444, -5.5947) knots 0 0 0 0 1 1 1 1
  spline S255 degree 3 poles (47.8444, -5.5947) (46.9674, -4.5997) (46.9674, -4.5997) (45.5942, -4.6083) knots 0 0 0 0 1 1 1 1
  spline S256 degree 3 poles (45.5942, -4.6083) (45.2178, -4.649) (44.8414, -4.6897) (44.4536, -4.7316) knots 0 0 0 0 1 1 1 1
  spline S257 degree 3 poles (21.766, 48.0419) (23.7394, 45.2001) (23.3427, 42.4701) (22.7524, 39.1641) knots 0 0 0 0 1 1 1 1
  spline S258 degree 3 poles (22.7524, 39.1641) (21.9305, 36.863) (20.9231, 35.4918) (18.8067, 34.232) knots 0 0 0 0 1 1 1 1
  spline S259 degree 3 poles (18.8067, 34.232) (17.4812, 34.2628) (17.4812, 34.2628) (16.3406, 34.7252) knots 0 0 0 0 1 1 1 1
  spline S260 degree 3 poles (16.3406, 34.7252) (14.7367, 37.1311) (14.7713, 39.0838) (15.2001, 41.8768) knots 0 0 0 0 1 1 1 1
  spline S261 degree 3 poles (15.2001, 41.8768) (15.668, 44.2132) (16.2887, 45.73) (17.8203, 47.5487) knots 0 0 0 0 1 1 1 1
  spline S262 degree 3 poles (17.8203, 47.5487) (19.1563, 48.2167) (20.2909, 48.074) (21.766, 48.0419) knots 0 0 0 0 1 1 1 1
  spline S263 degree 3 poles (-0.4285, 46.5623) (0.2498, 44.6782) (-0.0633, 43.0727) (-0.4285, 41.137) knots 0 0 0 0 1 1 1 1
  spline S264 degree 3 poles (-0.4285, 41.137) (-0.9217, 40.6437) (-0.9217, 40.6437) (-1.833, 40.5956) knots 0 0 0 0 1 1 1 1
  spline S265 degree 3 poles (-1.833, 40.5956) (-2.8445, 40.6116) (-3.8559, 40.6277) (-4.8674, 40.6437) knots 0 0 0 0 1 1 1 1
  spline S266 degree 3 poles (-4.8674, 40.6437) (-3.6114, 43.0162) (-2.4061, 44.7494) (-0.4285, 46.5623) knots 0 0 0 0 1 1 1 1
extrude "Extrude7" cut sketch "Sketch108" against normal blind 0.4 contours S4 S5 S6 S7 S8 S9 S10 S11 S12 S13 S14 S15 S16 S17 S18 S19 S20 S21 S22 | S23 S24 S25 S26 S27 S28 S29 S30 S31 S32 S33 S34 S35 S36 S37 S38 S39 S40 S41 S42 | S43 S44 S45 S46 S47 S48 S49 S50 S51 S52 S53 S54 S55 S56 S57 S58 S59 S60 S61 | S62 S63 S64 S65 S66 S67 S68 S69 | S70 S71 S72 S73 S74 S75 | S76 S77 S78 S79 S80 S81 S82 S83 S84 S85 S86 S87 S88 S89 S90 S91 S92 S93 S94 S95 S96 S97 S98 S99 S100 S101 S102 S103 S104 S105 S106 S107 S108 | S109 S110 S111 S112 S113 S114 S115 S116 S117 S118 S119 S120 S121 S122 S123 S124 S125 S126 S127 S128 S129 S130 S131 S132 S133 S134 S135 S136 S137 S138 S139 S140 S141 S142 S143 S144 S145 S146 S147 S148 S149 S150 S151 S152 S153 S154 S155 | S156 S157 S158 S159 S160 S161 S162 S163 S164 S165 S166 S167 S168 S169 S170 S171 S172 S173 S174 S175 S176 S177 S178 S179 S180 S181 S182 | S183 S184 S185 S186 S187 S188 S189 S190 S191 S192 S193 S194 S195 S196 S197 S198 S199 S200 S201 S202 S203 S204 S205 S206 S207 S208 S209 S210 S211 S212 S213 S214 S215 S216 | S217 S218 S219 S220 S221 S222 S223 S224 S225 S226 S227 S228 S229 S230 S231 S232 S233 S234 S235 S236 S237 S238 S239 S240 S241 S242 S243 S244 S245 S246 S247 S248 S249 S250 | S251 S252 S253 S254 S255 S256 bodies 2 in component "Component"
sketch "Sketch109" plane through (76.6406, 0, 0) normal (1, 0, 0) x (0, 1, 0)
  arc A0 (-52.887, 113.3681) -> (-58.3648, 106.1458) centre (-50.8648, 106.1458) ccw
  line L0 (-58.3648, 106.1458) -> (-58.3648, 16.8343)
  line L1 (-58.3648, 16.8343) -> (66.6352, 16.8343)
  line L2 (66.6352, 16.8343) -> (66.6352, 140.242)
  arc A1 (66.6352, 140.242) -> (60.2871, 145.0568) centre (61.6352, 140.242) ccw
  line L3 (60.2871, 145.0568) -> (-52.887, 113.3681)
sketch "Sketch110" plane through (76.6406, 0, 0) normal (1, 0, 0) x (0, 1, 0)
sketch "Sketch111" plane through (-103.3594, 0, 0) normal (-1, 0, 0) x (0, -1, 0)
  arc A0 (58.3648, 106.1458) -> (52.887, 113.3681) centre (50.8648, 106.1458) ccw
  line L0 (52.887, 113.3681) -> (-60.2871, 145.0568)
  arc A1 (-60.2871, 145.0568) -> (-66.6352, 140.242) centre (-61.6352, 140.242) ccw
  line L1 (-66.6352, 140.242) -> (-66.6352, 16.8343)
  line L2 (-66.6352, 16.8343) -> (58.3648, 16.8343)
  line L3 (58.3648, 16.8343) -> (58.3648, 106.1458)
  circle A2 centre (0, 70) radius 42.5
  dimension "d186" = 85
  measures "d186" diameter of A2
extrude "Extrude8" cut sketch "Sketch111" against normal blind 0.4 contours A2 bodies 2 in component "Component"
sketch "Sketch112" plane through (76.6406, 0, 0) normal (1, 0, 0) x (0, 1, 0)
  circle A0 centre (0, 70) radius 42.5
  dimension "d189" = 85
  measures "d189" diameter of A0
extrude "Extrude9" cut sketch "Sketch112" against normal blind 0.4 bodies 2 in component "Component"
sketch "Sketch113" plane through (71.6406, 0, 0) normal (-1, 0, 0) x (0, -1, 0)
  line L0 (54.3648, 91) -> (54.3648, 39.3343)
  line L1 (57.3648, 39.3343) -> (57.3648, 91)
  line L2 (57.3648, 91) -> (54.3648, 91)
  line L3 (57.3648, 91) -> (54.3648, 91)
  line L4 (54.3648, 91) -> (54.3648, 105.5147)
  line L5 (54.3648, 105.5147) -> (57.3648, 105.5147)
  line L6 (57.3648, 105.5147) -> (57.3648, 91)
  constraint horizontal L3
  constraint vertical L4
  constraint horizontal L5
  constraint vertical L6
  constraint coincident L1.end L2.start
extrude "Extrude10" cut sketch "Sketch113" along normal blind 170 bodies 2 in component "Component"
sketch "Sketch114" plane through (-98.3594, 0, 0) normal (1, 0, 0) x (0, 1, 0)
  line L0 (-54.3648, 39.3343) -> (-54.3648, 19.769)
  arc A0 (-46.1173, 21.8343) -> (-54.3648, 19.769) centre (-46.1173, 4.3343) ccw
  line L1 (-46.1173, 21.8343) -> (-10.7755, 21.8343)
  arc A1 (-10.7755, 21.8343) -> (61.6142, 145.2419) centre (-112.3399, 164.3463) ccw
  arc A2 (61.6142, 145.2419) -> (60.2871, 145.0568) centre (61.6352, 140.242) ccw
  line L2 (60.2871, 145.0568) -> (26.4871, 135.5928)
  line L3 (26.4871, 135.5928) -> (27.8352, 130.778)
  line L4 (27.8352, 130.778) -> (-53.3648, 108.042)
  line L5 (-53.3648, 108.042) -> (-53.3648, 39.3343)
  line L6 (-53.3648, 39.3343) -> (-54.3648, 39.3343)
sketch "Sketch115" plane through (71.6406, 0, 0) normal (-1, 0, 0) x (0, -1, 0)
  line L0 (54.3648, 59.6271) -> (57.3648, 59.6271)
  line L1 (54.3648, 39.3343) -> (54.3648, 64.7338)
  line L2 (57.3648, 64.7338) -> (57.3648, 39.3343)
  line L3 (54.3648, 39.3343) -> (54.3648, 19.769)
  line L4 (57.3648, 59.6271) -> (57.3648, 19.7124)
  line L5 (57.3648, 19.7124) -> (54.3648, 19.7124)
sketch "Sketch116" plane through (71.6406, 0, 0) normal (-1, 0, 0) x (0, -1, 0)
  line L0 (53.3648, 108.042) -> (53.3648, 39.3343)
  line L1 (58.3648, 111.8343) -> (58.3648, 16.8343)
  line L2 (54.3648, 108.042) -> (54.3648, 57)
  line L3 (57.3648, 59.6271) -> (57.3648, 19.7124)
  line L4 (57.3648, 19.7124) -> (54.3648, 19.7124)
  line L5 (54.3648, 39.3343) -> (54.3648, 19.769)
  line L6 (54.3648, 39.3343) -> (54.3648, 64.7338)
  line L7 (57.3648, 64.7338) -> (57.3648, 39.3343)
  line L8 (57.3648, 39.3343) -> (57.3648, 91)
  line L9 (54.3648, 91) -> (54.3648, 39.3343)
  line L10 (54.3648, 105.5169) -> (57.3648, 105.5169)
  line L11 (57.3648, 105.5169) -> (57.3648, 19.7124)
  line L12 (57.3648, 19.7124) -> (54.3648, 19.7124)
  line L13 (54.3648, 19.7124) -> (54.3648, 105.5169)
  dimension "d194" = 1
  constraint parallel L0 L2
  constraint horizontal L10
  constraint vertical L11
  constraint horizontal L12
  constraint vertical L13
  constraint coincident L3.end L4.start
  constraint coincident L2 L10.start
  measures "d194" distance of L0 L2
extrude "Extrude11" cut sketch "Sketch116" along normal blind 171.6 and the other way blind 1.6 bodies 2 in component "Component"
sketch "Sketch117" plane through (71.6406, 0, 0) normal (-1, 0, 0) x (0, -1, 0)
move_body "Move21" bodies 3 to x (1, 0, 0) y (0, 1, 0) z (0, 0, 1) at (0, 60, 0)
move_body "Move22" bodies 4 to x (1, 0, 0) y (0, 1, 0) z (0, 0, 1) at (-18, 105, 43)
combine "Combine3" operation add target body 3 tool bodies 4
move_body "Move23" bodies 3 to x (1, 0, 0) y (0, 1, 0) z (0, 0, 1) at (0, 0, 20)
component "Component" placed x (1, 0, 0) y (0, 1, 0) z (0, 0, 1) at (0, 0, 0)
